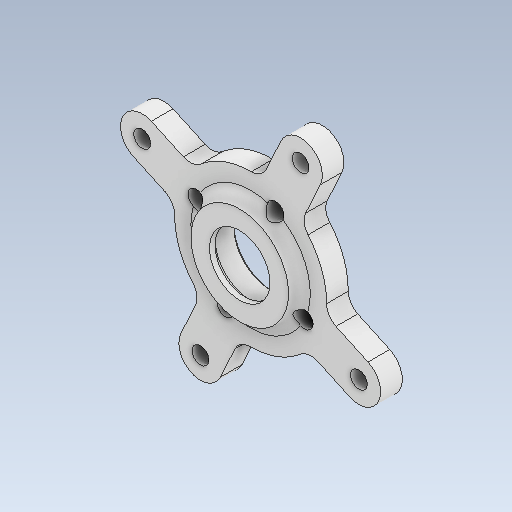
# Autodesk Inventor part: bearing_shell_2
Saved by Autodesk Inventor 2020 (Build 240168000, 168)
## iProperties
Created: 2020-07-17
Part Number: bearing_shell_2
Material: ABS Plastic
Document SubType Name: Modeling
Designer: psrobotics
Density: 1.06 g/cm^3
Appearance: Smooth - White
Author: psrobotics
Autodesk Inventor part; units mm, degrees
ref_plane "YZ Plane" through (0, 0, 0) normal (1, 0, 0) x (0, 1, 0)
ref_plane "XZ Plane" through (0, 0, 0) normal (0, 1, 0) x (-1, 0, 0)
ref_plane "XY Plane" through (0, 0, 0) normal (0, 0, 1) x (1, 0, 0)
sketch "Sketch1" plane through (0, 0, 0) normal (0, 0, 1) x (1, 0, 0)
  arc A0 (37.7593, 27.3905) -> (34.653, 36.1574) centre (-13.0849, 14.3094) ccw projected
  arc A1 (37.0904, 38.8916) -> (34.653, 36.1574) centre (36.4716, 36.9897) ccw projected
  arc A2 (37.0904, 38.8916) -> (41.8792, 38.064) centre (42.35, 55.0575) ccw projected
  arc A3 (43.7594, 35.5611) -> (41.8792, 38.064) centre (41.8238, 36.0648) ccw projected
  line L0 (43.7594, 35.5611) -> (41.6317, 27.3852) projected
  arc A4 (37.7593, 27.3905) -> (41.6317, 27.3852) centre (39.6962, 27.8889) ccw projected
  arc A5 (26.717, 61.7366) -> (25.3511, 54.8621) centre (42.35, 55.0575) ccw projected
  arc A6 (22.0141, 53.3517) -> (25.3511, 54.8621) centre (23.3512, 54.8391) ccw projected
  arc A7 (22.0141, 53.3517) -> (13.1352, 59.7929) centre (-13.0849, 14.3094) ccw projected
  arc A8 (13.9493, 63.5171) -> (13.1352, 59.7929) centre (14.1341, 61.5256) ccw projected
  line L1 (13.9493, 63.5171) -> (24.6931, 64.5138) projected
  arc A9 (26.717, 61.7366) -> (24.6931, 64.5138) centre (24.8778, 62.5224) ccw projected
  circle A10 centre (35.4446, 65.8812) radius 2.05 projected
  circle A11 centre (31.5263, 48.1521) radius 2.05 projected
  circle A12 centre (49.2554, 44.2339) radius 2.05 projected
  circle A13 centre (53.1736, 61.9629) radius 2.05 projected
  circle A14 centre (30.1445, 57.755) radius 1.55 projected
  circle A15 centre (54.5554, 52.36) radius 1.55 projected
  circle A16 centre (39.6525, 42.8521) radius 1.55 projected
  circle A17 centre (45.0475, 67.263) radius 1.55 projected
  line L2 (28.5807, -22.7664) -> (24.6864, -37.7313) projected
  arc A18 (21.1406, -38.4139) -> (24.6864, -37.7313) centre (22.7509, -37.2276) ccw projected
  arc A19 (21.1406, -38.4139) -> (18.5696, -35.453) centre (1.4153, -52.9453) ccw projected
  arc A20 (17.7668, -32.5556) -> (18.5696, -35.453) centre (20.6701, -33.3111) ccw projected
  line L3 (17.7668, -32.5556) -> (18.9871, -27.8663) projected
  arc A21 (20.5882, -25.3154) -> (18.9871, -27.8663) centre (23.826, -29.1255) ccw projected
  arc A22 (20.5882, -25.3154) -> (25.1737, -20.9082) centre (-13.0849, 14.3094) ccw projected
  arc A23 (28.5807, -22.7664) -> (25.1737, -20.9082) centre (26.6452, -22.2628) ccw projected
  arc A24 (-30.6719, -34.6263) -> (-23.8962, -36.5544) centre (-13.0849, 14.3094) ccw projected
  arc A25 (-22.5677, -39.4893) -> (-23.8962, -36.5544) centre (-24.312, -38.5107) ccw projected
  arc A26 (-22.5677, -39.4893) -> (-24.5732, -43.9538) centre (1.4153, -52.9453) ccw projected
  arc A27 (-28.0869, -44.4677) -> (-24.5732, -43.9538) centre (-26.4633, -43.2999) ccw projected
  line L4 (-28.0869, -44.4677) -> (-32.9719, -37.6763) projected
  arc A28 (-30.6719, -34.6263) -> (-32.9719, -37.6763) centre (-31.3483, -36.5085) ccw projected
  circle A29 centre (21.3872, -62.1714) radius 2.05 projected
  circle A30 centre (10.6414, -32.9733) radius 2.05 projected
  circle A31 centre (-18.5566, -43.7191) radius 2.05 projected
  circle A32 centre (-7.8109, -72.9172) radius 2.05 projected
  circle A33 centre (-6.1085, 26.3929) radius 2.1 projected
  circle A34 centre (-13.0849, 54.978) radius 2.1 projected
  circle A35 centre (-20.0614, 26.3929) radius 2.1 projected
  circle A36 centre (-48.305, 34.6437) radius 2.1 projected
  circle A37 centre (-27.0378, 14.3094) radius 2.1 projected
  circle A38 centre (-48.305, -6.025) radius 2.1 projected
  circle A39 centre (-20.0614, 2.2258) radius 2.1 projected
  circle A40 centre (-13.0849, -26.3593) radius 2.1 projected
  circle A41 centre (-6.1085, 2.2258) radius 2.1 projected
  circle A42 centre (22.1351, -6.025) radius 2.1 projected
  circle A43 centre (22.1351, 34.6437) radius 2.1 projected
  circle A44 centre (0.868, 14.3094) radius 2.1 projected
  line L5 (-6.6298, 35.0022) -> (-11.5528, 29.1352) projected
  arc A45 (-14.617, 29.1352) -> (-11.5528, 29.1352) centre (-13.0849, 30.4208) ccw projected
  line L6 (-14.617, 29.1352) -> (-19.54, 35.0022) projected
  arc A46 (-17.7841, 39.8812) -> (-19.54, 35.0022) centre (-17.2419, 36.9306) ccw projected
  arc A47 (-8.3858, 39.8812) -> (-17.7841, 39.8812) centre (-13.0849, 14.3094) ccw projected
  arc A48 (-6.6298, 35.0022) -> (-8.3858, 39.8812) centre (-8.928, 36.9306) ccw projected
  line L7 (-27.7779, 30.246) -> (-25.1585, 23.0491) projected
  arc A49 (-26.6905, 20.3955) -> (-25.1585, 23.0491) centre (-27.0378, 22.3651) ccw projected
  line L8 (-26.6905, 20.3955) -> (-34.233, 19.0655) projected
  arc A50 (-37.5803, 23.0257) -> (-34.233, 19.0655) centre (-34.7539, 22.0199) ccw projected
  arc A51 (-32.8812, 31.1649) -> (-37.5803, 23.0257) centre (-13.0849, 14.3094) ccw projected
  arc A52 (-27.7779, 30.246) -> (-32.8812, 31.1649) centre (-30.597, 29.22) ccw projected
  line L9 (-34.233, 9.5532) -> (-26.6905, 8.2232) projected
  arc A53 (-25.1585, 5.5696) -> (-26.6905, 8.2232) centre (-27.0378, 6.2536) ccw projected
  line L10 (-25.1585, 5.5696) -> (-27.7779, -1.6273) projected
  arc A54 (-32.8812, -2.5461) -> (-27.7779, -1.6273) centre (-30.597, -0.6013) ccw projected
  arc A55 (-37.5803, 5.593) -> (-32.8812, -2.5461) centre (-13.0849, 14.3094) ccw projected
  arc A56 (-34.233, 9.5532) -> (-37.5803, 5.593) centre (-34.7539, 6.5988) ccw projected
  line L11 (-19.54, -6.3835) -> (-14.617, -0.5165) projected
  arc A57 (-11.5528, -0.5165) -> (-14.617, -0.5165) centre (-13.0849, -1.8021) ccw projected
  line L12 (-11.5528, -0.5165) -> (-6.6298, -6.3835) projected
  arc A58 (-8.3858, -11.2625) -> (-6.6298, -6.3835) centre (-8.928, -8.3119) ccw projected
  arc A59 (-17.7841, -11.2625) -> (-8.3858, -11.2625) centre (-13.0849, 14.3094) ccw projected
  arc A60 (-19.54, -6.3835) -> (-17.7841, -11.2625) centre (-17.2419, -8.3119) ccw projected
  line L13 (1.6081, -1.6273) -> (-1.0114, 5.5696) projected
  arc A61 (0.5207, 8.2232) -> (-1.0114, 5.5696) centre (0.868, 6.2536) ccw projected
  line L14 (0.5207, 8.2232) -> (8.0632, 9.5532) projected
  arc A62 (11.4105, 5.593) -> (8.0632, 9.5532) centre (8.5841, 6.5988) ccw projected
  arc A63 (6.7113, -2.5461) -> (11.4105, 5.593) centre (-13.0849, 14.3094) ccw projected
  arc A64 (1.6081, -1.6273) -> (6.7113, -2.5461) centre (4.4272, -0.6013) ccw projected
  line L15 (8.0632, 19.0655) -> (0.5207, 20.3955) projected
  arc A65 (-1.0114, 23.0491) -> (0.5207, 20.3955) centre (0.868, 22.3651) ccw projected
  line L16 (-1.0114, 23.0491) -> (1.6081, 30.246) projected
  arc A66 (6.7113, 31.1649) -> (1.6081, 30.246) centre (4.4272, 29.22) ccw projected
  arc A67 (11.4105, 23.0257) -> (6.7113, 31.1649) centre (-13.0849, 14.3094) ccw projected
  arc A68 (8.0632, 19.0655) -> (11.4105, 23.0257) centre (8.5841, 22.0199) ccw projected
  arc A69 (-45.9141, -17.9124) -> (-24.5752, -30.2325) centre (-13.0849, 14.3094) ccw projected
  arc A70 (-45.5767, -12.002) -> (-45.9141, -17.9124) centre (-43.0594, -15.1105) ccw projected
  line L17 (-45.5767, -12.002) -> (-40.5749, -7.9516) projected
  arc A71 (-36.5234, -8.2048) -> (-40.5749, -7.9516) centre (-38.687, -10.283) ccw projected
  arc A72 (-36.5234, -8.2048) -> (-20.8635, -17.246) centre (-13.0849, 14.3094) ccw projected
  arc A73 (-18.6185, -20.6282) -> (-20.8635, -17.246) centre (-21.5815, -20.1589) ccw projected
  line L18 (-18.6185, -20.6282) -> (-19.6253, -26.985) projected
  arc A74 (-24.5752, -30.2325) -> (-19.6253, -26.985) centre (-23.5761, -26.3593) ccw projected
  arc A75 (-1.5946, -30.2325) -> (19.7443, -17.9124) centre (-13.0849, 14.3094) ccw projected
  arc A76 (-6.5445, -26.985) -> (-1.5946, -30.2325) centre (-2.5938, -26.3593) ccw projected
  line L19 (-6.5445, -26.985) -> (-7.5514, -20.6282) projected
  arc A77 (-5.3063, -17.246) -> (-7.5514, -20.6282) centre (-4.5883, -20.1589) ccw projected
  arc A78 (-5.3063, -17.246) -> (10.3536, -8.2048) centre (-13.0849, 14.3094) ccw projected
  arc A79 (14.4051, -7.9516) -> (10.3536, -8.2048) centre (12.5171, -10.283) ccw projected
  line L20 (14.4051, -7.9516) -> (19.4068, -12.002) projected
  arc A80 (19.7443, -17.9124) -> (19.4068, -12.002) centre (16.8896, -15.1105) ccw projected
  arc A81 (31.2346, 1.9893) -> (31.2346, 26.6294) centre (-13.0849, 14.3094) ccw projected
  arc A82 (25.9472, -0.6737) -> (31.2346, 1.9893) centre (27.3807, 3.0606) ccw projected
  line L21 (25.9472, -0.6737) -> (19.9386, 1.6328) projected
  arc A83 (18.1322, 5.2681) -> (19.9386, 1.6328) centre (21.0137, 4.4335) ccw projected
  arc A84 (18.1322, 5.2681) -> (18.1322, 23.3506) centre (-13.0849, 14.3094) ccw projected
  arc A85 (19.9386, 26.9859) -> (18.1322, 23.3506) centre (21.0137, 24.1852) ccw projected
  line L22 (19.9386, 26.9859) -> (25.9472, 29.2924) projected
  arc A86 (31.2346, 26.6294) -> (25.9472, 29.2924) centre (27.3807, 25.5581) ccw projected
  arc A87 (19.7443, 46.5311) -> (-1.5946, 58.8512) centre (-13.0849, 14.3094) ccw projected
  arc A88 (19.4068, 40.6207) -> (19.7443, 46.5311) centre (16.8896, 43.7293) ccw projected
  line L23 (19.4068, 40.6207) -> (14.4051, 36.5703) projected
  arc A89 (10.3536, 36.8235) -> (14.4051, 36.5703) centre (12.5171, 38.9017) ccw projected
  arc A90 (10.3536, 36.8235) -> (-5.3063, 45.8648) centre (-13.0849, 14.3094) ccw projected
  arc A91 (-7.5514, 49.2469) -> (-5.3063, 45.8648) centre (-4.5883, 48.7776) ccw projected
  line L24 (-7.5514, 49.2469) -> (-6.5445, 55.6037) projected
  arc A92 (-1.5946, 58.8512) -> (-6.5445, 55.6037) centre (-2.5938, 54.978) ccw projected
  arc A93 (-24.5752, 58.8512) -> (-45.9141, 46.5311) centre (-13.0849, 14.3094) ccw projected
  arc A94 (-19.6253, 55.6037) -> (-24.5752, 58.8512) centre (-23.5761, 54.978) ccw projected
  line L25 (-19.6253, 55.6037) -> (-18.6185, 49.2469) projected
  arc A95 (-20.8635, 45.8648) -> (-18.6185, 49.2469) centre (-21.5815, 48.7776) ccw projected
  arc A96 (-20.8635, 45.8648) -> (-36.5234, 36.8235) centre (-13.0849, 14.3094) ccw projected
  arc A97 (-40.5749, 36.5703) -> (-36.5234, 36.8235) centre (-38.687, 38.9017) ccw projected
  line L26 (-40.5749, 36.5703) -> (-45.5767, 40.6207) projected
  arc A98 (-45.9141, 46.5311) -> (-45.5767, 40.6207) centre (-43.0594, 43.7293) ccw projected
  arc A99 (-57.4044, 26.6294) -> (-57.4044, 1.9893) centre (-13.0849, 14.3094) ccw projected
  arc A100 (-52.1171, 29.2924) -> (-57.4044, 26.6294) centre (-53.5505, 25.5581) ccw projected
  line L27 (-52.1171, 29.2924) -> (-46.1085, 26.9859) projected
  arc A101 (-44.302, 23.3506) -> (-46.1085, 26.9859) centre (-47.1836, 24.1852) ccw projected
  arc A102 (-44.302, 23.3506) -> (-44.302, 5.2681) centre (-13.0849, 14.3094) ccw projected
  arc A103 (-46.1085, 1.6328) -> (-44.302, 5.2681) centre (-47.1836, 4.4335) ccw projected
  line L28 (-46.1085, 1.6328) -> (-52.1171, -0.6737) projected
  arc A104 (-57.4044, 1.9893) -> (-52.1171, -0.6737) centre (-53.5505, 3.0606) ccw projected
  circle A105 centre (1.4153, -52.9453) radius 16 projected
  circle A106 centre (-13.0849, 14.3094) radius 8 projected
  circle A107 centre (42.35, 55.0575) radius 8 projected
  circle A108 centre (11.4314, -80.1607) radius 1.5 projected
  circle A109 centre (-67.4662, 1.2099) radius 1.5 projected
  circle A110 centre (-64.6648, 36.8793) radius 1.5 projected
  circle A111 centre (51.8859, 79.5742) radius 1.5 projected
  circle A112 centre (50.8041, 30.1471) radius 1.5 projected
  circle A113 centre (68.6496, 55.6331) radius 1.5 projected
  circle A114 centre (21.8333, 71.5216) radius 1.5 projected
  circle A115 centre (-53.6308, 52.8444) radius 1.5 projected
  circle A116 centre (-69.0394, 20.5532) radius 1.5 projected
  circle A117 centre (-15.8701, -76.5718) radius 1.5 projected
  circle A118 centre (29.8929, -59.7296) radius 1.5 projected
  line L29 (27.7736, -49.6922) -> (47.1491, 24.7628) projected
  arc A119 (48.7374, 26.2287) -> (47.1491, 24.7628) centre (49.0847, 24.2591) ccw projected
  line L30 (48.7374, 26.2287) -> (55.3511, 27.3949) projected
  line L31 (55.3511, 27.3949) -> (54.9554, 29.6389) projected
  arc A120 (55.9198, 31.7153) -> (54.9554, 29.6389) centre (56.925, 29.9862) ccw projected
  arc A121 (55.9198, 31.7153) -> (68.9256, 50.2896) centre (42.35, 55.0575) ccw projected
  arc A122 (70.5469, 51.906) -> (68.9256, 50.2896) centre (70.8942, 49.9364) ccw projected
  line L32 (70.5469, 51.906) -> (72.791, 52.3017) projected
  line L33 (72.791, 52.3017) -> (71.4018, 60.1801) projected
  line L34 (71.4018, 60.1801) -> (66.3972, 59.2977) projected
  arc A123 (64.1152, 60.7604) -> (66.3972, 59.2977) centre (66.0499, 61.2673) ccw projected
  arc A124 (64.1152, 60.7604) -> (55.1531, 73.5597) centre (42.35, 55.0575) ccw projected
  arc A125 (54.5591, 76.2043) -> (55.1531, 73.5597) centre (56.2911, 75.2043) ccw projected
  line L35 (54.5591, 76.2043) -> (57.1, 80.6053) projected
  line L36 (57.1, 80.6053) -> (50.1718, 84.6053) projected
  line L37 (50.1718, 84.6053) -> (49.0324, 82.6319) projected
  arc A126 (46.959, 81.6612) -> (49.0324, 82.6319) centre (47.3004, 83.6319) ccw projected
  arc A127 (46.959, 81.6612) -> (25.0566, 75.7925) centre (42.35, 55.0575) ccw projected
  arc A128 (22.7756, 75.5964) -> (25.0566, 75.7925) centre (23.7756, 77.3284) ccw projected
  line L38 (22.7756, 75.5964) -> (20.8022, 76.7357) projected
  line L39 (20.8022, 76.7357) -> (17.3195, 70.7034) projected
  arc A129 (15.7722, 69.712) -> (17.3195, 70.7034) centre (15.5874, 71.7034) ccw projected
  line L40 (15.7722, 69.712) -> (-17.9347, 66.5849) projected
  arc A130 (-17.9347, 66.5849) -> (-37.6487, 60.7084) centre (-13.0849, 14.3094) ccw projected
  arc A131 (-40.3166, 61.4759) -> (-37.6487, 60.7084) centre (-38.5845, 62.4759) ccw projected
  line L41 (-40.3166, 61.4759) -> (-42.8712, 65.9007) projected
  line L42 (-42.8712, 65.9007) -> (-55.4508, 55.9968) projected
  arc A132 (-55.4508, 55.9968) -> (-58.9228, 52.1458) centre (-13.0849, 14.3094) ccw projected
  line L43 (-58.9228, 52.1458) -> (-58.1742, 51.5278) projected
  arc A133 (-57.8623, 48.7657) -> (-58.1742, 51.5278) centre (-59.4473, 49.9854) ccw projected
  arc A134 (-57.8623, 48.7657) -> (-62.6354, 41.4571) centre (-13.0849, 14.3094) ccw projected
  arc A135 (-65.2899, 40.6322) -> (-62.6354, 41.4571) centre (-64.3894, 42.4181) ccw projected
  line L44 (-65.2899, 40.6322) -> (-66.4827, 41.2337) projected
  arc A136 (-66.4827, 41.2337) -> (-69.0046, 35.5046) centre (-13.0849, 14.3094) ccw projected
  line L45 (-69.0046, 35.5046) -> (-72.1104, 23.9135) projected
  arc A137 (-72.1104, 23.9135) -> (-72.791, 17.6911) centre (-13.0849, 14.3094) ccw projected
  line L46 (-72.791, 17.6911) -> (-71.4572, 17.6155) projected
  arc A138 (-69.5708, 15.574) -> (-71.4572, 17.6155) centre (-71.5703, 15.6187) ccw projected
  arc A139 (-69.5708, 15.574) -> (-69.0914, 6.858) centre (-13.0849, 14.3094) ccw projected
  arc A140 (-70.7426, 4.6219) -> (-69.0914, 6.858) centre (-71.0739, 6.5942) ccw projected
  line L47 (-70.7426, 4.6219) -> (-71.6999, 4.461) projected
  arc A141 (-71.6999, 4.461) -> (-70.6186, -0.6102) centre (-13.0849, 14.3094) ccw projected
  line L48 (-70.6186, -0.6102) -> (-64.6763, -15.4769) projected
  line L49 (-64.6763, -15.4769) -> (-60.2515, -12.9223) projected
  arc A142 (-57.5573, -13.5915) -> (-60.2515, -12.9223) centre (-59.2515, -14.6543) ccw projected
  arc A143 (-57.5573, -13.5915) -> (-55.7049, -16.3465) centre (-13.0849, 14.3094) ccw projected
  line L50 (-55.7049, -16.3465) -> (-19.1732, -67.1356) projected
  arc A144 (-19.7312, -74.8103) -> (-19.1732, -67.1356) centre (-24.0441, -70.6391) ccw projected
  line L51 (-19.7312, -74.8103) -> (-21.5262, -76.6663) projected
  line L52 (-21.5262, -76.6663) -> (-17.2133, -80.8375) projected
  line L53 (-17.2133, -80.8375) -> (-14.3852, -80.7903) projected
  line L54 (-14.3852, -80.7903) -> (-12.8656, -79.219) projected
  arc A145 (-10.5858, -78.7953) -> (-12.8656, -79.219) centre (-11.4279, -80.6093) ccw projected
  arc A146 (-10.5858, -78.7953) -> (5.8048, -81.1052) centre (1.4153, -52.9453) ccw projected
  arc A147 (7.9898, -82.3906) -> (5.8048, -81.1052) centre (6.1129, -83.0813) ccw projected
  line L55 (7.9898, -82.3906) -> (8.3683, -83.4191) projected
  line L56 (8.3683, -83.4191) -> (10.936, -84.6053) projected
  line L57 (10.936, -84.6053) -> (14.6898, -83.2237) projected
  line L58 (14.6898, -83.2237) -> (15.876, -80.6561) projected
  line L59 (15.876, -80.6561) -> (15.4975, -79.6275) projected
  arc A148 (16.3279, -77.2324) -> (15.4975, -79.6275) centre (17.3744, -78.9367) ccw projected
  arc A149 (16.3279, -77.2324) -> (27.3106, -64.8483) centre (1.4153, -52.9453) ccw projected
  arc A150 (29.3212, -63.6929) -> (27.3106, -64.8483) centre (29.1278, -65.6836) ccw projected
  line L60 (29.3212, -63.6929) -> (31.4969, -63.9042) projected
  line L61 (31.4969, -63.9042) -> (33.6808, -62.1069) projected
  line L62 (33.6808, -62.1069) -> (34.2608, -56.135) projected
  line L63 (34.2608, -56.135) -> (32.1292, -55.928) projected
  arc A151 (27.7736, -49.6922) -> (32.1292, -55.928) centre (32.6125, -50.9514) ccw projected
  circle A152 centre (1.4153, -52.9453) radius 6.575
  circle A153 centre (1.4153, -52.9453) radius 14
  point P0 (0, 0)
  dimension "d0" = 13.15
  dimension "d1" = 28
  constraints: 2 centre point, 2 coincident
  measures "d0" diameter of A152
  measures "d1" diameter of A153
extrude "Extrusion1" add sketch "Sketch1" along normal blind 4 contours A153
sketch "Sketch2" plane through (1.4153, -52.9453, 4) normal (0, 0, 1) x (1, 0, 0)
  arc A0 (36.344, 80.3358) -> (33.2377, 89.1027) centre (-14.5002, 67.2546) ccw projected
  arc A1 (35.6751, 91.8369) -> (33.2377, 89.1027) centre (35.0563, 89.935) ccw projected
  arc A2 (35.6751, 91.8369) -> (40.4639, 91.0093) centre (40.9347, 108.0028) ccw projected
  arc A3 (42.3441, 88.5064) -> (40.4639, 91.0093) centre (40.4085, 89.0101) ccw projected
  line L0 (42.3441, 88.5064) -> (40.2164, 80.3304) projected
  arc A4 (36.344, 80.3358) -> (40.2164, 80.3304) centre (38.2809, 80.8341) ccw projected
  arc A5 (25.3017, 114.6819) -> (23.9358, 107.8073) centre (40.9347, 108.0028) ccw projected
  arc A6 (20.5988, 106.297) -> (23.9358, 107.8073) centre (21.9359, 107.7843) ccw projected
  arc A7 (20.5988, 106.297) -> (11.7199, 112.7382) centre (-14.5002, 67.2546) ccw projected
  arc A8 (12.534, 116.4624) -> (11.7199, 112.7382) centre (12.7188, 114.4709) ccw projected
  line L1 (12.534, 116.4624) -> (23.2778, 117.4591) projected
  arc A9 (25.3017, 114.6819) -> (23.2778, 117.4591) centre (23.4625, 115.4676) ccw projected
  circle A10 centre (34.0293, 118.8264) radius 2.05 projected
  circle A11 centre (30.111, 101.0974) radius 2.05 projected
  circle A12 centre (47.8401, 97.1791) radius 2.05 projected
  circle A13 centre (51.7583, 114.9082) radius 2.05 projected
  circle A14 centre (28.7292, 110.7003) radius 1.55 projected
  circle A15 centre (53.1401, 105.3053) radius 1.55 projected
  circle A16 centre (38.2372, 95.7973) radius 1.55 projected
  circle A17 centre (43.6322, 120.2083) radius 1.55 projected
  line L2 (27.1654, 30.1788) -> (23.2711, 15.2139) projected
  arc A18 (19.7253, 14.5314) -> (23.2711, 15.2139) centre (21.3356, 15.7176) ccw projected
  arc A19 (19.7253, 14.5314) -> (17.1543, 17.4923) centre (0, 0) ccw projected
  arc A20 (16.3515, 20.3897) -> (17.1543, 17.4923) centre (19.2548, 19.6342) ccw projected
  line L3 (16.3515, 20.3897) -> (17.5718, 25.079) projected
  arc A21 (19.1729, 27.6298) -> (17.5718, 25.079) centre (22.4107, 23.8198) ccw projected
  arc A22 (19.1729, 27.6298) -> (23.7584, 32.037) centre (-14.5002, 67.2546) ccw projected
  arc A23 (27.1654, 30.1788) -> (23.7584, 32.037) centre (25.2299, 30.6825) ccw projected
  arc A24 (-32.0872, 18.319) -> (-25.3114, 16.3909) centre (-14.5002, 67.2546) ccw projected
  arc A25 (-23.983, 13.456) -> (-25.3114, 16.3909) centre (-25.7273, 14.4346) ccw projected
  arc A26 (-23.983, 13.456) -> (-25.9885, 8.9914) centre (0, 0) ccw projected
  arc A27 (-29.5022, 8.4775) -> (-25.9885, 8.9914) centre (-27.8786, 9.6454) ccw projected
  line L4 (-29.5022, 8.4775) -> (-34.3872, 15.269) projected
  arc A28 (-32.0872, 18.319) -> (-34.3872, 15.269) centre (-32.7636, 16.4368) ccw projected
  circle A29 centre (19.9719, -9.2261) radius 2.05 projected
  circle A30 centre (9.2261, 19.9719) radius 2.05 projected
  circle A31 centre (-19.9719, 9.2261) radius 2.05 projected
  circle A32 centre (-9.2261, -19.9719) radius 2.05 projected
  circle A33 centre (-7.5238, 79.3382) radius 2.1 projected
  circle A34 centre (-14.5002, 107.9232) radius 2.1 projected
  circle A35 centre (-21.4767, 79.3382) radius 2.1 projected
  circle A36 centre (-49.7203, 87.5889) radius 2.1 projected
  circle A37 centre (-28.4531, 67.2546) radius 2.1 projected
  circle A38 centre (-49.7203, 46.9203) radius 2.1 projected
  circle A39 centre (-21.4767, 55.171) radius 2.1 projected
  circle A40 centre (-14.5002, 26.586) radius 2.1 projected
  circle A41 centre (-7.5238, 55.171) radius 2.1 projected
  circle A42 centre (20.7198, 46.9203) radius 2.1 projected
  circle A43 centre (20.7198, 87.5889) radius 2.1 projected
  circle A44 centre (-0.5473, 67.2546) radius 2.1 projected
  line L5 (-8.0451, 87.9475) -> (-12.9681, 82.0805) projected
  arc A45 (-16.0323, 82.0805) -> (-12.9681, 82.0805) centre (-14.5002, 83.3661) ccw projected
  line L6 (-16.0323, 82.0805) -> (-20.9553, 87.9475) projected
  arc A46 (-19.1994, 92.8264) -> (-20.9553, 87.9475) centre (-18.6572, 89.8758) ccw projected
  arc A47 (-9.8011, 92.8264) -> (-19.1994, 92.8264) centre (-14.5002, 67.2546) ccw projected
  arc A48 (-8.0451, 87.9475) -> (-9.8011, 92.8264) centre (-10.3433, 89.8758) ccw projected
  line L7 (-29.1932, 83.1913) -> (-26.5738, 75.9944) projected
  arc A49 (-28.1058, 73.3407) -> (-26.5738, 75.9944) centre (-28.4531, 75.3103) ccw projected
  line L8 (-28.1058, 73.3407) -> (-35.6483, 72.0108) projected
  arc A50 (-38.9956, 75.9709) -> (-35.6483, 72.0108) centre (-36.1692, 74.9652) ccw projected
  arc A51 (-34.2965, 84.1101) -> (-38.9956, 75.9709) centre (-14.5002, 67.2546) ccw projected
  arc A52 (-29.1932, 83.1913) -> (-34.2965, 84.1101) centre (-32.0123, 82.1653) ccw projected
  line L9 (-35.6483, 62.4984) -> (-28.1058, 61.1685) projected
  arc A53 (-26.5738, 58.5149) -> (-28.1058, 61.1685) centre (-28.4531, 59.1989) ccw projected
  line L10 (-26.5738, 58.5149) -> (-29.1932, 51.3179) projected
  arc A54 (-34.2965, 50.3991) -> (-29.1932, 51.3179) centre (-32.0123, 52.344) ccw projected
  arc A55 (-38.9956, 58.5383) -> (-34.2965, 50.3991) centre (-14.5002, 67.2546) ccw projected
  arc A56 (-35.6483, 62.4984) -> (-38.9956, 58.5383) centre (-36.1692, 59.544) ccw projected
  line L11 (-20.9553, 46.5618) -> (-16.0323, 52.4287) projected
  arc A57 (-12.9681, 52.4287) -> (-16.0323, 52.4287) centre (-14.5002, 51.1432) ccw projected
  line L12 (-12.9681, 52.4287) -> (-8.0451, 46.5618) projected
  arc A58 (-9.8011, 41.6828) -> (-8.0451, 46.5618) centre (-10.3433, 44.6334) ccw projected
  arc A59 (-19.1994, 41.6828) -> (-9.8011, 41.6828) centre (-14.5002, 67.2546) ccw projected
  arc A60 (-20.9553, 46.5618) -> (-19.1994, 41.6828) centre (-18.6572, 44.6334) ccw projected
  line L13 (0.1928, 51.3179) -> (-2.4267, 58.5149) projected
  arc A61 (-0.8946, 61.1685) -> (-2.4267, 58.5149) centre (-0.5473, 59.1989) ccw projected
  line L14 (-0.8946, 61.1685) -> (6.6479, 62.4984) projected
  arc A62 (9.9952, 58.5383) -> (6.6479, 62.4984) centre (7.1688, 59.544) ccw projected
  arc A63 (5.2961, 50.3991) -> (9.9952, 58.5383) centre (-14.5002, 67.2546) ccw projected
  arc A64 (0.1928, 51.3179) -> (5.2961, 50.3991) centre (3.0119, 52.344) ccw projected
  line L15 (6.6479, 72.0108) -> (-0.8946, 73.3407) projected
  arc A65 (-2.4267, 75.9944) -> (-0.8946, 73.3407) centre (-0.5473, 75.3103) ccw projected
  line L16 (-2.4267, 75.9944) -> (0.1928, 83.1913) projected
  arc A66 (5.2961, 84.1101) -> (0.1928, 83.1913) centre (3.0119, 82.1653) ccw projected
  arc A67 (9.9952, 75.9709) -> (5.2961, 84.1101) centre (-14.5002, 67.2546) ccw projected
  arc A68 (6.6479, 72.0108) -> (9.9952, 75.9709) centre (7.1688, 74.9652) ccw projected
  arc A69 (-47.3294, 35.0328) -> (-25.9905, 22.7128) centre (-14.5002, 67.2546) ccw projected
  arc A70 (-46.992, 40.9433) -> (-47.3294, 35.0328) centre (-44.4747, 37.8347) ccw projected
  line L17 (-46.992, 40.9433) -> (-41.9902, 44.9937) projected
  arc A71 (-37.9387, 44.7405) -> (-41.9902, 44.9937) centre (-40.1022, 42.6622) ccw projected
  arc A72 (-37.9387, 44.7405) -> (-22.2788, 35.6992) centre (-14.5002, 67.2546) ccw projected
  arc A73 (-20.0338, 32.3171) -> (-22.2788, 35.6992) centre (-22.9968, 32.7864) ccw projected
  line L18 (-20.0338, 32.3171) -> (-21.0406, 25.9603) projected
  arc A74 (-25.9905, 22.7128) -> (-21.0406, 25.9603) centre (-24.9914, 26.586) ccw projected
  arc A75 (-3.0099, 22.7128) -> (18.329, 35.0328) centre (-14.5002, 67.2546) ccw projected
  arc A76 (-7.9598, 25.9603) -> (-3.0099, 22.7128) centre (-4.0091, 26.586) ccw projected
  line L19 (-7.9598, 25.9603) -> (-8.9667, 32.3171) projected
  arc A77 (-6.7216, 35.6992) -> (-8.9667, 32.3171) centre (-6.0036, 32.7864) ccw projected
  arc A78 (-6.7216, 35.6992) -> (8.9383, 44.7405) centre (-14.5002, 67.2546) ccw projected
  arc A79 (12.9898, 44.9937) -> (8.9383, 44.7405) centre (11.1018, 42.6622) ccw projected
  line L20 (12.9898, 44.9937) -> (17.9916, 40.9433) projected
  arc A80 (18.329, 35.0328) -> (17.9916, 40.9433) centre (15.4743, 37.8347) ccw projected
  arc A81 (29.8193, 54.9346) -> (29.8193, 79.5746) centre (-14.5002, 67.2546) ccw projected
  arc A82 (24.5319, 52.2716) -> (29.8193, 54.9346) centre (25.9654, 56.0059) ccw projected
  line L21 (24.5319, 52.2716) -> (18.5233, 54.5781) projected
  arc A83 (16.7169, 58.2134) -> (18.5233, 54.5781) centre (19.5984, 57.3788) ccw projected
  arc A84 (16.7169, 58.2134) -> (16.7169, 76.2959) centre (-14.5002, 67.2546) ccw projected
  arc A85 (18.5233, 79.9312) -> (16.7169, 76.2959) centre (19.5984, 77.1304) ccw projected
  line L22 (18.5233, 79.9312) -> (24.5319, 82.2377) projected
  arc A86 (29.8193, 79.5746) -> (24.5319, 82.2377) centre (25.9654, 78.5033) ccw projected
  arc A87 (18.329, 99.4764) -> (-3.0099, 111.7964) centre (-14.5002, 67.2546) ccw projected
  arc A88 (17.9916, 93.5659) -> (18.329, 99.4764) centre (15.4743, 96.6745) ccw projected
  line L23 (17.9916, 93.5659) -> (12.9898, 89.5156) projected
  arc A89 (8.9383, 89.7688) -> (12.9898, 89.5156) centre (11.1018, 91.847) ccw projected
  arc A90 (8.9383, 89.7688) -> (-6.7216, 98.81) centre (-14.5002, 67.2546) ccw projected
  arc A91 (-8.9667, 102.1921) -> (-6.7216, 98.81) centre (-6.0036, 101.7228) ccw projected
  line L24 (-8.9667, 102.1921) -> (-7.9598, 108.549) projected
  arc A92 (-3.0099, 111.7964) -> (-7.9598, 108.549) centre (-4.0091, 107.9232) ccw projected
  arc A93 (-25.9905, 111.7964) -> (-47.3294, 99.4764) centre (-14.5002, 67.2546) ccw projected
  arc A94 (-21.0406, 108.549) -> (-25.9905, 111.7964) centre (-24.9914, 107.9232) ccw projected
  line L25 (-21.0406, 108.549) -> (-20.0338, 102.1921) projected
  arc A95 (-22.2788, 98.81) -> (-20.0338, 102.1921) centre (-22.9968, 101.7228) ccw projected
  arc A96 (-22.2788, 98.81) -> (-37.9387, 89.7688) centre (-14.5002, 67.2546) ccw projected
  arc A97 (-41.9902, 89.5156) -> (-37.9387, 89.7688) centre (-40.1022, 91.847) ccw projected
  line L26 (-41.9902, 89.5156) -> (-46.992, 93.5659) projected
  arc A98 (-47.3294, 99.4764) -> (-46.992, 93.5659) centre (-44.4747, 96.6745) ccw projected
  arc A99 (-58.8197, 79.5746) -> (-58.8197, 54.9346) centre (-14.5002, 67.2546) ccw projected
  arc A100 (-53.5324, 82.2377) -> (-58.8197, 79.5746) centre (-54.9658, 78.5033) ccw projected
  line L27 (-53.5324, 82.2377) -> (-47.5238, 79.9312) projected
  arc A101 (-45.7173, 76.2959) -> (-47.5238, 79.9312) centre (-48.5989, 77.1304) ccw projected
  arc A102 (-45.7173, 76.2959) -> (-45.7173, 58.2134) centre (-14.5002, 67.2546) ccw projected
  arc A103 (-47.5238, 54.5781) -> (-45.7173, 58.2134) centre (-48.5989, 57.3788) ccw projected
  line L28 (-47.5238, 54.5781) -> (-53.5324, 52.2716) projected
  arc A104 (-58.8197, 54.9346) -> (-53.5324, 52.2716) centre (-54.9658, 56.0059) ccw projected
  circle A105 centre (0, 0) radius 16 projected
  circle A106 centre (-14.5002, 67.2546) radius 8 projected
  circle A107 centre (40.9347, 108.0028) radius 8 projected
  circle A108 centre (10.0161, -27.2154) radius 1.5 projected
  circle A109 centre (-68.8815, 54.1552) radius 1.5 projected
  circle A110 centre (-66.0801, 89.8245) radius 1.5 projected
  circle A111 centre (50.4706, 132.5195) radius 1.5 projected
  circle A112 centre (49.3888, 83.0924) radius 1.5 projected
  circle A113 centre (67.2343, 108.5784) radius 1.5 projected
  circle A114 centre (20.418, 124.4669) radius 1.5 projected
  circle A115 centre (-55.0461, 105.7897) radius 1.5 projected
  circle A116 centre (-70.4547, 73.4984) radius 1.5 projected
  circle A117 centre (-17.2854, -23.6266) radius 1.5 projected
  circle A118 centre (28.4776, -6.7844) radius 1.5 projected
  line L29 (26.3583, 3.2531) -> (45.7338, 77.7081) projected
  arc A119 (47.3221, 79.174) -> (45.7338, 77.7081) centre (47.6694, 77.2044) ccw projected
  line L30 (47.3221, 79.174) -> (53.9358, 80.3401) projected
  line L31 (53.9358, 80.3401) -> (53.5401, 82.5842) projected
  arc A120 (54.5045, 84.6606) -> (53.5401, 82.5842) centre (55.5097, 82.9315) ccw projected
  arc A121 (54.5045, 84.6606) -> (67.5103, 103.2348) centre (40.9347, 108.0028) ccw projected
  arc A122 (69.1316, 104.8513) -> (67.5103, 103.2348) centre (69.4789, 102.8816) ccw projected
  line L32 (69.1316, 104.8513) -> (71.3757, 105.2469) projected
  line L33 (71.3757, 105.2469) -> (69.9865, 113.1254) projected
  line L34 (69.9865, 113.1254) -> (64.9819, 112.243) projected
  arc A123 (62.6999, 113.7057) -> (64.9819, 112.243) centre (64.6346, 114.2126) ccw projected
  arc A124 (62.6999, 113.7057) -> (53.7378, 126.505) centre (40.9347, 108.0028) ccw projected
  arc A125 (53.1438, 129.1496) -> (53.7378, 126.505) centre (54.8758, 128.1496) ccw projected
  line L35 (53.1438, 129.1496) -> (55.6847, 133.5505) projected
  line L36 (55.6847, 133.5505) -> (48.7565, 137.5505) projected
  line L37 (48.7565, 137.5505) -> (47.6171, 135.5771) projected
  arc A126 (45.5437, 134.6065) -> (47.6171, 135.5771) centre (45.8851, 136.5771) ccw projected
  arc A127 (45.5437, 134.6065) -> (23.6413, 128.7378) centre (40.9347, 108.0028) ccw projected
  arc A128 (21.3603, 128.5417) -> (23.6413, 128.7378) centre (22.3603, 130.2737) ccw projected
  line L38 (21.3603, 128.5417) -> (19.3869, 129.681) projected
  line L39 (19.3869, 129.681) -> (15.9042, 123.6487) projected
  arc A129 (14.3569, 122.6572) -> (15.9042, 123.6487) centre (14.1721, 124.6487) ccw projected
  line L40 (14.3569, 122.6572) -> (-19.35, 119.5301) projected
  arc A130 (-19.35, 119.5301) -> (-39.064, 113.6536) centre (-14.5002, 67.2546) ccw projected
  arc A131 (-41.7319, 114.4212) -> (-39.064, 113.6536) centre (-39.9998, 115.4212) ccw projected
  line L41 (-41.7319, 114.4212) -> (-44.2865, 118.846) projected
  line L42 (-44.2865, 118.846) -> (-56.8661, 108.9421) projected
  arc A132 (-56.8661, 108.9421) -> (-60.3381, 105.091) centre (-14.5002, 67.2546) ccw projected
  line L43 (-60.3381, 105.091) -> (-59.5894, 104.473) projected
  arc A133 (-59.2776, 101.7109) -> (-59.5894, 104.473) centre (-60.8626, 102.9306) ccw projected
  arc A134 (-59.2776, 101.7109) -> (-64.0507, 94.4024) centre (-14.5002, 67.2546) ccw projected
  arc A135 (-66.7052, 93.5775) -> (-64.0507, 94.4024) centre (-65.8047, 95.3633) ccw projected
  line L44 (-66.7052, 93.5775) -> (-67.898, 94.179) projected
  arc A136 (-67.898, 94.179) -> (-70.4199, 88.4499) centre (-14.5002, 67.2546) ccw projected
  line L45 (-70.4199, 88.4499) -> (-73.5257, 76.8588) projected
  arc A137 (-73.5257, 76.8588) -> (-74.2063, 70.6363) centre (-14.5002, 67.2546) ccw projected
  line L46 (-74.2063, 70.6363) -> (-72.8725, 70.5608) projected
  arc A138 (-70.9861, 68.5192) -> (-72.8725, 70.5608) centre (-72.9856, 68.564) ccw projected
  arc A139 (-70.9861, 68.5192) -> (-70.5067, 59.8033) centre (-14.5002, 67.2546) ccw projected
  arc A140 (-72.1578, 57.5671) -> (-70.5067, 59.8033) centre (-72.4892, 59.5395) ccw projected
  line L47 (-72.1578, 57.5671) -> (-73.1152, 57.4063) projected
  arc A141 (-73.1152, 57.4063) -> (-72.0339, 52.3351) centre (-14.5002, 67.2546) ccw projected
  line L48 (-72.0339, 52.3351) -> (-66.0915, 37.4683) projected
  line L49 (-66.0915, 37.4683) -> (-61.6668, 40.023) projected
  arc A142 (-58.9726, 39.3538) -> (-61.6668, 40.023) centre (-60.6668, 38.2909) ccw projected
  arc A143 (-58.9726, 39.3538) -> (-57.1202, 36.5987) centre (-14.5002, 67.2546) ccw projected
  line L50 (-57.1202, 36.5987) -> (-20.5885, -14.1903) projected
  arc A144 (-21.1465, -21.865) -> (-20.5885, -14.1903) centre (-25.4594, -17.6939) ccw projected
  line L51 (-21.1465, -21.865) -> (-22.9415, -23.7211) projected
  line L52 (-22.9415, -23.7211) -> (-18.6286, -27.8922) projected
  line L53 (-18.6286, -27.8922) -> (-15.8005, -27.845) projected
  line L54 (-15.8005, -27.845) -> (-14.2809, -26.2737) projected
  arc A145 (-12.0011, -25.85) -> (-14.2809, -26.2737) centre (-12.8432, -27.6641) ccw projected
  arc A146 (-12.0011, -25.85) -> (4.3895, -28.1599) centre (0, 0) ccw projected
  arc A147 (6.5745, -29.4453) -> (4.3895, -28.1599) centre (4.6976, -30.1361) ccw projected
  line L55 (6.5745, -29.4453) -> (6.953, -30.4739) projected
  line L56 (6.953, -30.4739) -> (9.5207, -31.66) projected
  line L57 (9.5207, -31.66) -> (13.2746, -30.2785) projected
  line L58 (13.2746, -30.2785) -> (14.4607, -27.7108) projected
  line L59 (14.4607, -27.7108) -> (14.0822, -26.6822) projected
  arc A148 (14.9126, -24.2871) -> (14.0822, -26.6822) centre (15.9591, -25.9915) ccw projected
  arc A149 (14.9126, -24.2871) -> (25.8953, -11.903) centre (0, 0) ccw projected
  arc A150 (27.9059, -10.7477) -> (25.8953, -11.903) centre (27.7125, -12.7383) ccw projected
  line L60 (27.9059, -10.7477) -> (30.0816, -10.959) projected
  line L61 (30.0816, -10.959) -> (32.2655, -9.1617) projected
  line L62 (32.2655, -9.1617) -> (32.8455, -3.1898) projected
  line L63 (32.8455, -3.1898) -> (30.7139, -2.9827) projected
  arc A151 (26.3583, 3.2531) -> (30.7139, -2.9827) centre (31.1972, 1.9938) ccw projected
  circle A152 centre (0, 0) radius 14 projected
  circle A153 centre (0, 0) radius 6.575 projected
  circle A154 centre (19.9719, -9.2261) radius 4
  line L64 (19.9719, -9.2261) -> (0, 0)
  line L65 (19.9719, -9.2261) -> (0, 0) construction
  line L66 (21.6494, -5.5949) -> (1.6775, 3.6313)
  line L67 (-1.6775, -3.6313) -> (18.2945, -12.8574)
  arc A155 (18.2945, -12.8574) -> (21.6494, -5.5949) centre (19.9719, -9.2261) ccw
  arc A156 (1.6775, 3.6313) -> (-1.6775, -3.6313) centre (0, 0) ccw
  point P0 (-1.4153, 52.9453)
  point P1 (9.986, -4.6131)
  point P2 (21.6494, -5.5949)
  point P3 (13.8571, -1.9952)
  point P4 (10.5021, -9.2577)
  point P5 (18.2945, -12.8574)
  dimension "d4" = 8
  dimension "d5" = 8
  constraints: 10 end point, 4 point on circle, 4 tangent, 3 centre point, 2 equal length, 1 coincident, 1 midpoint
  measures "d4" diameter of A154
  measures "d5" diameter of A156
extrude "Extrusion2" add sketch "Sketch2" against normal blind 4 contours A29 | L67 A152 L64 A105 | A105 L64 A154 L67 | L66 A154 L64 A105 | A105 L64 A152 L66 | A154
pattern_circular "Circular Pattern1" count 4 over 360 about axis through (1.4153, -52.9453, 0) along (0, 0, 1) of "Extrusion2"
sketch "Sketch3" plane through (0, 0, 4) normal (0, 0, 1) x (1, 0, 0)
  arc A0 (15.2724, -54.9404) -> (10.673, -42.4431) centre (1.4153, -52.9453) ccw projected
  line L0 (10.673, -42.4431) -> (14.2727, -34.6508) projected
  arc A1 (14.2727, -34.6508) -> (7.0102, -31.2958) centre (10.6414, -32.9733) ccw projected
  line L1 (7.0102, -31.2958) -> (3.4105, -39.0882) projected
  arc A2 (3.4105, -39.0882) -> (-9.0868, -43.6876) centre (1.4153, -52.9453) ccw projected
  line L2 (-9.0868, -43.6876) -> (-16.8792, -40.0879) projected
  arc A3 (-16.8792, -40.0879) -> (-20.2341, -47.3504) centre (-18.5566, -43.7191) ccw projected
  line L3 (-20.2341, -47.3504) -> (-12.4418, -50.9501) projected
  arc A4 (-12.4418, -50.9501) -> (-7.8424, -63.4474) centre (1.4153, -52.9453) ccw projected
  line L4 (-7.8424, -63.4474) -> (-11.4421, -71.2397) projected
  arc A5 (-11.4421, -71.2397) -> (-4.1796, -74.5947) centre (-7.8109, -72.9172) ccw projected
  line L5 (-4.1796, -74.5947) -> (-0.5799, -66.8024) projected
  arc A6 (-0.5799, -66.8024) -> (11.9174, -62.203) centre (1.4153, -52.9453) ccw projected
  line L6 (11.9174, -62.203) -> (19.7097, -65.8027) projected
  arc A7 (19.7097, -65.8027) -> (23.0647, -58.5402) centre (21.3872, -62.1714) ccw projected
  line L7 (23.0647, -58.5402) -> (15.2724, -54.9404) projected
  circle A8 centre (1.4153, -52.9453) radius 6.575 projected
  point P0 (0, 0)
hole "Hole1" at (21.3872, -62.1714, 4) at (-7.8109, -72.9172, 4) at (-18.5566, -43.7191, 4) at (10.6414, -32.9733, 4) direction (0, 0, -1) diameter 3.1 depth 17
fillet "Fillet1" radius 3 8 edges at (15.2724, -54.9404, 2) (11.9174, -62.203, 2) (-0.5799, -66.8024, 2) (-7.8424, -63.4474, 2) (-12.4418, -50.9501, 2) (-9.0868, -43.6876, 2) (3.4105, -39.0882, 2) (10.673, -42.4431, 2)
sketch "Sketch4" plane through (0, 0, 4) normal (0, 0, 1) x (1, 0, 0)
  circle A0 centre (-18.5566, -43.7191) radius 1.55 projected
  circle A1 centre (21.3872, -62.1714) radius 1.55 projected
  circle A2 centre (-7.8109, -72.9172) radius 1.55 projected
  circle A3 centre (10.6414, -32.9733) radius 1.55 projected
  arc A4 (15.4148, -53.0623) -> (11.9989, -43.7808) centre (1.4153, -52.9453) ccw projected
  arc A5 (11.5434, -40.5589) -> (11.9989, -43.7808) centre (14.2669, -41.817) ccw projected
  line L0 (11.5434, -40.5589) -> (14.2727, -34.6508) projected
  arc A6 (14.2727, -34.6508) -> (7.0102, -31.2958) centre (10.6414, -32.9733) ccw projected
  line L1 (7.0102, -31.2958) -> (4.2809, -37.204) projected
  arc A7 (1.5324, -38.9458) -> (4.2809, -37.204) centre (1.5574, -35.9459) ccw projected
  arc A8 (1.5324, -38.9458) -> (-7.7491, -42.3616) centre (1.4153, -52.9453) ccw projected
  arc A9 (-10.971, -42.8171) -> (-7.7491, -42.3616) centre (-9.7129, -40.0937) ccw projected
  line L2 (-10.971, -42.8171) -> (-16.8792, -40.0879) projected
  arc A10 (-16.8792, -40.0879) -> (-20.2341, -47.3504) centre (-18.5566, -43.7191) ccw projected
  line L3 (-20.2341, -47.3504) -> (-14.326, -50.0797) projected
  arc A11 (-12.5842, -52.8282) -> (-14.326, -50.0797) centre (-15.5841, -52.8031) ccw projected
  arc A12 (-12.5842, -52.8282) -> (-9.1683, -62.1097) centre (1.4153, -52.9453) ccw projected
  arc A13 (-8.7128, -65.3316) -> (-9.1683, -62.1097) centre (-11.4363, -64.0735) ccw projected
  line L4 (-8.7128, -65.3316) -> (-11.4421, -71.2397) projected
  arc A14 (-11.4421, -71.2397) -> (-4.1796, -74.5947) centre (-7.8109, -72.9172) ccw projected
  line L5 (-4.1796, -74.5947) -> (-1.4503, -68.6866) projected
  arc A15 (1.2982, -66.9448) -> (-1.4503, -68.6866) centre (1.2731, -69.9447) ccw projected
  arc A16 (1.2982, -66.9448) -> (10.5797, -63.5289) centre (1.4153, -52.9453) ccw projected
  arc A17 (13.8016, -63.0734) -> (10.5797, -63.5289) centre (12.5435, -65.7968) ccw projected
  line L6 (13.8016, -63.0734) -> (19.7097, -65.8027) projected
  arc A18 (19.7097, -65.8027) -> (23.0647, -58.5402) centre (21.3872, -62.1714) ccw projected
  line L7 (23.0647, -58.5402) -> (17.1566, -55.8109) projected
  arc A19 (15.4148, -53.0623) -> (17.1566, -55.8109) centre (18.4147, -53.0874) ccw projected
  circle A20 centre (1.4153, -52.9453) radius 6.575 projected
  line L8 (1.4153, -52.9453) -> (21.3872, -62.1714)
  line L9 (1.4153, -52.9453) -> (11.4013, -57.5583)
  circle A21 centre (11.4013, -57.5583) radius 1.55
  point P0 (0, 0)
  dimension "d19" = 11
  dimension "d20" = 3.1
  constraints: 4 end point, 2 coincident, 1 centre point, 1 midpoint
  measures "d19" distance of L9.start L9.end
  measures "d20" diameter of A21
extrude "Extrusion3" cut sketch "Sketch4" against normal blind 4 contours A21 L8 | L8 A21
pattern_circular "Circular Pattern2" count 4 over 360 about axis through (1.4153, -52.9453, 0) along (0, 0, 1) of "Extrusion3"
sketch "Sketch5" plane through (0, 0, 4) normal (0, 0, 1) x (1, 0, 0)
  circle A0 centre (1.4153, -52.9453) radius 6.575 projected
  circle A1 centre (1.4153, -52.9453) radius 9
  circle A2 centre (1.4153, -52.9453) radius 5.575
  point P0 (0, 0)
  dimension "d29" = 18
  dimension "d30" = 1
  constraints: 2 centre point, 2 coincident
  measures "d29" diameter of A1
  measures "d30" radial gap between concentric circles of A0 A2
extrude "Extrusion4" add sketch "Sketch5" along normal blind 2 contours A0 | A1
chamfer "Chamfer2" distance 1 angle 45 1 edges at (-4.1597, -52.9453, 4)
chamfer "Chamfer3" distance 0.5 angle 45 1 edges at (-5.1597, -52.9453, 0)
fillet "Fillet2" radius 2 1 edges at (-7.5847, -52.9453, 4)
body "Solid1"
